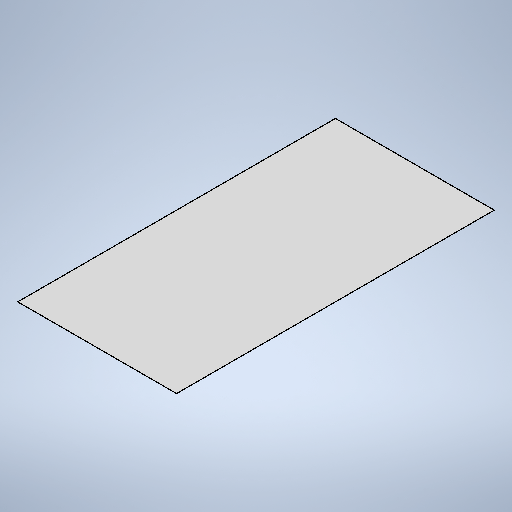
# Autodesk Inventor part: PNS-0111 floor sheet 1
Saved by Autodesk Inventor 2025 (Build 290162010, 162A)
## iProperties
Created: 2025-03-10
Part Number: PNS-0111 floor sheet 1
Material: Stainless Steel
Description: DIE16(5)|\ 90°|corrY -___°|X_____|bom___
Document SubType Name: Sheet Metal
Designer: admin
Stock Number: МОО 305 шпангоут борт
Mass: 50000 g
Surface Area: 62650 cm^2
Volume: 6250 cm^3
Density: 8 g/cm^3
Sheet Metal Rule: AISI304 2mm Die16
Sheet Metal Width: 1250,000 mm
Sheet Metal Length: 2500,000 mm
Sheet Metal Area: 3125000,000 mm^2
Appearance: Default
Flat Pattern Width: 125 cm
Flat Pattern Length: 250 cm
Flat Pattern Area: 31250 cm^2
Author: admin
Autodesk Inventor part; units mm, degrees
ref_plane "YZ Plane" through (0, 0, 0) normal (1, 0, 0) x (0, 1, 0)
ref_plane "XZ Plane" through (0, 0, 0) normal (0, 1, 0) x (-1, 0, 0)
ref_plane "XY Plane" through (0, 0, 0) normal (0, 0, 1) x (1, 0, 0)
sketch "Sketch1" plane through (0, 0, 0) normal (0, 0, 1) x (1, 0, 0)
  line L0 (-625, -1250) -> (625, -1250)
  line L1 (625, -1250) -> (625, 1250)
  line L2 (625, 1250) -> (-625, 1250)
  line L3 (-625, 1250) -> (-625, -1250)
  line L4 (-625, -1250) -> (625, 1250) construction
  line L5 (625, -1250) -> (-625, 1250) construction
  point P0 (0, 0)
  dimension "d154" = 1250
  dimension "d155" = 2500
  measures "d154" distance of L1.end L2.end
  measures "d155" distance of L0.end L1.end
extrude "Plate5" add sketch "Sketch1" along normal blind 2
body "Solid3"
